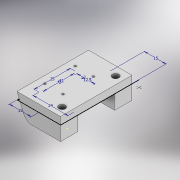
# Autodesk Inventor part: camera_holder
Saved by Autodesk Inventor 2021 (Build 250183000, 183)
## iProperties
Created: 2020-07-28
Part Number: camera_holder
Material: Generic
Document SubType Name: Modeling
Designer: Mazur
Density: 1 g/cm^3
Appearance: Default
Author: Mazur
Autodesk Inventor part; units mm, degrees
ref_plane "YZ Plane" through (0, 0, 0) normal (1, 0, 0) x (0, 1, 0)
ref_plane "XZ Plane" through (0, 0, 0) normal (0, 1, 0) x (-1, 0, 0)
ref_plane "XY Plane" through (0, 0, 0) normal (0, 0, 1) x (1, 0, 0)
sketch "Sketch1" plane through (0, 0, 0) normal (0, 1, 0) x (-1, 0, 0)
  circle A0 centre (9.758, -6.2456) radius 2.1174
  circle A1 centre (9.758, -6.2456) radius 2.1174
  circle A2 centre (9.758, -43.1772) radius 2.1174
  circle A3 centre (9.758, -43.1772) radius 2.1174
  line L0 (19.6065, 0) -> (19.6065, -49.3325)
  line L1 (19.6065, 0) -> (4.6065, 0)
  line L2 (4.6065, 0) -> (4.6065, -49.3325)
  line L3 (4.6065, -49.3325) -> (19.6065, -49.3325)
  line L4 (19.6065, -49.3325) -> (19.6065, 0)
  line L5 (4.6065, -49.3325) -> (4.6065, -54.3325)
  line L6 (19.6065, -49.3325) -> (34.6065, -49.3325)
  line L7 (34.6065, -49.3325) -> (34.6065, 0)
  line L8 (34.6065, 0) -> (19.6065, 0)
  line L9 (19.6065, 0) -> (19.6065, -49.3325)
  line L10 (34.6065, 0) -> (4.6065, -49.3325)
  line L11 (34.6065, -49.3325) -> (4.6065, 0)
  line L12 (7.6065, -37.1662) -> (31.6065, -37.1662)
  line L13 (31.6065, -37.1662) -> (31.6065, -12.1662)
  line L14 (31.6065, -12.1662) -> (7.6065, -12.1662)
  line L15 (7.6065, -12.1662) -> (7.6065, -37.1662)
  line L16 (7.6065, -37.1662) -> (31.6065, -12.1662) construction
  line L17 (31.6065, -37.1662) -> (7.6065, -12.1662) construction
  line L18 (17.1065, -14.1662) -> (29.6065, -14.1662)
  line L19 (29.6065, -14.1662) -> (29.6065, -35.1662)
  line L20 (29.6065, -35.1662) -> (17.1065, -35.1662)
  line L21 (17.1065, -35.1662) -> (17.1065, -14.1662)
  point P0 (0, 0)
  point P1 (19.6065, -49.3325)
  point P2 (-0.0904, -49.3325)
  point P3 (19.6065, -24.6662)
  dimension "d0" = 15
  dimension "d5" = 15
  dimension "d8" = 24
  dimension "d9" = 25
  dimension "d14" = 12.5
  dimension "d15" = 21
  dimension "d16" = 2
  dimension "d17" = 2
  constraints: 44 end point, 8 parallel, 4 centre point, 4 horizontal, 4 perpendicular, 3 midpoint, 2 coincident
  measures "d0" distance between parallel lines of L4 L2
  measures "d5" distance of L8.end L7.end
  measures "d8" distance of L14.end L13.end
  measures "d9" distance of L13.end L12.end
  measures "d14" distance of L19.end L20.end
  measures "d15" distance of L18.end L19.end
  measures "d16" distance between parallel lines of L12 L20
  measures "d17" distance between parallel lines of L13 L19
extrude "Extrusion1" add sketch "Sketch1" along normal blind 5 contours A0 L11 L1 L0 L14 | A0 L11 L14 L15 L12 L10 A2 L2 | L14 L0 L18 L21 L11 | L11 L21 L10 L12 L15 L14 | L8 L10 L14 L0 | L10 A2 L12 L0 L3 | L21 L18 L0 L11 | L11 L10 L21 | L14 L10 L18 L0 | L7 L11 L12 L13 L14 L10 | L0 L12 L11 L6 | L11 L20 L0 | L0 L18 L10 | L0 L20 L21 L10 | L10 L18 L19 L20 L11 | L21 L20 L0 L12 L10 | L14 L13 L12 L11 L20 L19 L18 L10 | L0 L20 L11 L12
hole "Hole1" at (0.0904, 0, -49.3325) at (-29.6065, 0, -35.1662) at (-29.6065, 0, -14.1662) at (-17.1065, 0, -35.1662) at (-17.1065, 0, -14.1662) direction (0, 1, 0) diameter 1.5 end through all
sketch "Sketch2" plane through (0, 0, 0) normal (0, -1, 0) x (1, 0, 0)
  line L0 (-4.6065, 0) -> (-34.6065, 0)
  line L1 (-34.6065, 0) -> (-34.6065, -12)
  line L2 (-34.6065, -12) -> (-4.6065, -12)
  line L3 (-4.6065, -12) -> (-4.6065, 0)
  line L4 (-4.6065, -49.3325) -> (-34.6065, -49.3325)
  line L5 (-34.6065, -49.3325) -> (-34.6065, -37.3325)
  line L6 (-34.6065, -37.3325) -> (-4.6065, -37.3325)
  line L7 (-4.6065, -37.3325) -> (-4.6065, -49.3325)
  point P0 (0, 0)
  dimension "d27" = 30
  dimension "d28" = 12
  dimension "d29" = 30
  dimension "d30" = 12
  constraints: 16 end point, 4 parallel, 2 horizontal, 2 perpendicular
  measures "d27" distance of L2.end L1.end
  measures "d28" distance of L1.end L0.end
  measures "d29" distance of L5.end L6.end
  measures "d30" distance of L4.end L5.end
extrude "Extrusion2" add sketch "Sketch2" along normal blind 10
hole "Hole2" at (-9.758, 0, -6.2456) at (-9.758, 0, -43.1772) direction (0, -1, 0) diameter 4.5 end through all both
chamfer "Chamfer1" distance 8 angle 45 2 edges at (-34.6065, -10, -43.3325) (-34.6065, -10, -6)
chamfer "Chamfer2" distance 7 angle 45 2 edges at (-34.6065, -2, -43.3325) (-34.6065, -2, -6)
fillet "Fillet1" radius 4 4 edges at (-29.6574, -6.949, -6) (-26.6065, -10, -6) (-26.6065, -10, -43.3325) (-29.6574, -6.949, -43.3325)
body "Solid1"
